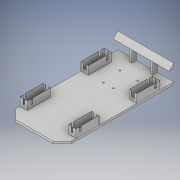
# Autodesk Inventor part: RC Chassis
Saved by Autodesk Inventor 2019 (Build 230136000, 136)
## iProperties
Created: 2020-11-23
Part Number: RC Chassis
Material: Generic
Document SubType Name: Modeling
Designer: wrong
Density: 1 g/cm^3
Appearance: Default
Author: wrong
Autodesk Inventor part; units mm, degrees
ref_plane "YZ Plane" through (0, 0, 0) normal (1, 0, 0) x (0, 1, 0)
sketch "Sketch1" plane through (0, 0, 0) normal (0, 1, 0) x (-1, 0, 0)
  line L0 (0, 0) -> (152.4, 0)
  line L1 (152.4, 0) -> (152.4, 304.8)
  line L2 (152.4, 304.8) -> (0, 304.8)
  line L3 (0, 304.8) -> (0, 0)
  dimension "d0" = 152.4
  dimension "d1" = 304.8
  constraints: 8 end point, 2 parallel, 1 horizontal, 1 perpendicular
  measures "d0" distance of L2.end L1.end
  measures "d1" distance of L1.end L0.end
extrude "Extrusion1" add sketch "Sketch1" along normal blind 50.8
sketch "Sketch3" plane through (0, 50.8, 0) normal (0, 1, 0) x (1, 0, 0)
  line L0 (-152.4, -12.7) -> (0, -12.7)
  line L1 (0, -12.7) -> (0, -304.8)
  line L2 (0, -304.8) -> (-152.4, -304.8)
  line L3 (-152.4, -304.8) -> (-152.4, -12.7)
  line L4 (0, 0) -> (-152.4, 0) projected
  line L5 (0, -304.8) -> (0, 0) projected
  dimension "d8" = 12.7
  dimension "d9" = 152.4
  dimension "d10" = 0
  dimension "d11" = 292.1
  constraints: 8 end point, 2 parallel, 1 horizontal, 1 perpendicular
  measures "d8" distance between parallel lines of L4 L0
  measures "d9" distance of L1.end L2.end
  measures "d10" distance between parallel lines of L5 L1
  measures "d11" distance of L2.end L0.start
extrude "Extrusion2" cut sketch "Sketch3" against normal blind 44.45
sketch "Sketch4" plane through (-152.4, 50.8, 12.7) normal (0, 0, 1) x (1, 0, 0)
  line L0 (10.16, -44.45) -> (0, -44.45)
  line L1 (107.95, -12.7) -> (101.6, -12.7)
  line L2 (101.6, -12.7) -> (101.6, -44.45)
  line L3 (101.6, -44.45) -> (107.95, -44.45)
  line L4 (107.95, -44.45) -> (107.95, -12.7)
  line L5 (152.4, 0) -> (152.4, -44.45) projected
  line L6 (0, 0) -> (152.4, 0) projected
  line L7 (152.4, -44.45) -> (0, -44.45) projected
  line L8 (44.45, -12.7) -> (50.8, -12.7)
  line L9 (50.8, -12.7) -> (50.8, -44.45)
  line L10 (50.8, -44.45) -> (44.45, -44.45)
  line L11 (44.45, -44.45) -> (44.45, -12.7)
  line L12 (0, -44.45) -> (0, 0) projected
  line L13 (44.45, -12.7) -> (0, -12.7)
  line L14 (44.45, -12.7) -> (152.4, -12.7)
  point P0 (152.4, -50.8)
  dimension "d15" = 44.45
  dimension "d16" = 6.35
  dimension "d18" = 31.75
  dimension "d22" = 0
  dimension "d23" = 6.35
  dimension "d24" = 31.75
  dimension "d25" = 44.45
  constraints: 22 end point, 4 parallel, 4 point on line, 3 horizontal, 2 perpendicular
  measures "d15" distance between parallel lines of L5 L4
  measures "d16" distance of L1.start L1.end
  measures "d18" distance of L1.end L2.end
  measures "d22" distance between parallel lines of L7 L3
  measures "d23" distance of L8.start L8.end
  measures "d24" distance of L10.end L8.start
  measures "d25" distance between parallel lines of L12 L11
extrude "Extrusion3" cut sketch "Sketch4" against normal through all contours L0 L12 L13 L11 L7 | L9 L14 L2 L7 | L4 L14 L5 L7
chamfer "Chamfer1" distance 12.7 angle 45 1 edges at (-76.2, 50.8, 12.7)
chamfer "Chamfer2" distance 25.4 angle 45 2 edges at (-152.4, 3.175, 304.8) (0, 3.175, 304.8) measured on face at (-101.6, 2.1167, 304.8)
sketch "Sketch8" plane through (0, 6.35, 0) normal (0, 1, 0) x (1, 0, 0)
  line L0 (-102.7176, -33.0495) -> (-49.7078, -33.0495)
  line L1 (-49.7078, -33.0495) -> (-49.7078, -100.3087)
  line L2 (-49.7078, -100.3087) -> (-102.7176, -100.3087)
  line L3 (-102.7176, -100.3087) -> (-102.7176, -33.0495)
  circle A0 centre (-94.0562, -97.3877) radius 1.9939
  circle A1 centre (-67.056, -97.3877) radius 1.9939
  circle A2 centre (-100.5078, -46.4861) radius 1.9939
  circle A3 centre (-51.9176, -46.4861) radius 1.9939
  line L4 (-25.3492, -49.0474) -> (-25.3492, -97.3582) projected
  line L5 (-67.056, -97.3877) -> (-51.9176, -97.3877)
  point P0 (0, 0)
  dimension "d72" = 53.0098
  dimension "d73" = 67.2592
  dimension "d74" = 3.9878
  dimension "d75" = 2.921
  dimension "d76" = 8.6614
  dimension "d77" = 3.9878
  dimension "d78" = 27.0002
  dimension "d79" = 3.9878
  dimension "d81" = 2.2098
  dimension "d84" = 3.9878
  dimension "d85" = 2.2098
  dimension "d87" = 24.3586
  dimension "d99" = 50.9016
  dimension "d100" = 13.4366
  dimension "d101" = 13.4366
  constraints: 10 end point, 4 centre point, 2 horizontal, 2 parallel, 1 perpendicular
  measures "d72" distance of L1.end L2.end
  measures "d73" distance of L0.end L1.end
  measures "d74" diameter of A0
  measures "d75" distance from line of L2 A0.centre
  measures "d76" distance from line of L3 A0.centre
  measures "d77" diameter of A1
  measures "d78" distance of L5.start A0.centre
  measures "d79" diameter of A2
  measures "d81" distance from line of L3 A2.centre
  measures "d84" diameter of A3
  measures "d85" distance from line of L1 A3.centre
  measures "d87" distance between parallel lines of L1 L4
  measures "d99" distance from line of A3.centre L5
  measures "d100" distance from line of L0 A3.centre
  measures "d101" distance from line of L0 A2.centre
hole "Hole1" at (-94.0562, 6.35, 97.3877) at (-67.056, 6.35, 97.3877) at (-100.5078, 6.35, 46.4861) at (-51.9176, 6.35, 46.4861) direction (0, -1, 0) diameter 3.9878 end through all
sketch "Sketch11" plane through (0, 6.35, 0) normal (0, 1, 0) x (1, 0, 0)
  line L0 (-143.515, -33.715) -> (-143.515, -38.215) projected
  line L1 (-141.015, -33.715) -> (-141.015, -38.215) projected
  line L2 (-143.515, -33.215) -> (-141.015, -33.215) projected
  line L3 (-142.265, -75.215) -> (-133.265, -75.215) projected
  line L4 (-133.265, -75.215) -> (-133.265, -43.215) projected
  line L5 (-133.265, -43.215) -> (-151.265, -43.215) projected
  line L6 (-151.265, -43.215) -> (-151.265, -75.215) projected
  line L7 (-151.265, -75.215) -> (-142.265, -75.215) projected
  line L8 (-151.265, -38.215) -> (-133.265, -38.215) projected
  line L9 (-160.765, -52.415) -> (-123.765, -52.415)
  line L10 (-160.765, -47.015) -> (-123.765, -47.015)
  line L11 (-150.565, -75.215) -> (-150.565, -86.215) projected
  line L12 (-149.165, -100.215) -> (-143.2099, -100.215) projected
  line L13 (-141.3201, -100.215) -> (-135.365, -100.215) projected
  line L14 (-146.165, -102.415) -> (-137.365, -102.415) projected
  arc A0 (-132.765, -38.715) -> (-133.265, -38.215) centre (-133.265, -38.715) ccw projected
  arc A1 (-151.265, -38.215) -> (-151.765, -38.715) centre (-151.265, -38.715) ccw projected
  line L15 (-151.765, -38.715) -> (-151.765, -43.215) projected
  line L16 (-132.765, -43.215) -> (-132.765, -38.715) projected
  line L17 (-143.015, -103.215) -> (-141.515, -103.215) projected
  line L18 (-152.019, -37.961) -> (-132.511, -37.961)
  line L19 (-132.511, -37.961) -> (-132.511, -100.469)
  line L20 (-132.511, -100.469) -> (-152.019, -100.469)
  line L21 (-152.019, -100.469) -> (-152.019, -37.961)
  line L22 (-152.4, -279.4) -> (-152.4, 0) projected
  line L23 (-152.4, -37.58) -> (-132.13, -37.58)
  line L24 (-132.13, -37.58) -> (-132.13, -100.85)
  line L25 (-132.13, -100.85) -> (-152.4, -100.85)
  line L26 (-152.4, -100.85) -> (-152.4, -37.58)
  line L27 (-76.2, -26.595) -> (-76.2, -134.8867)
  line L28 (0, 0) -> (0, -279.4) projected
  line L29 (-19.889, -37.961) -> (-19.889, -100.469)
  dimension "d102" = 0.254
  dimension "d103" = 0.254
  dimension "d104" = 0.254
  dimension "d105" = 0.254
  dimension "d106" = 0.381
  dimension "d107" = 0.381
  dimension "d108" = 0.381
  dimension "d115" = 76.2
  constraints: 24 end point, 4 horizontal, 4 parallel, 2 perpendicular, 2 symmetric about line, 1 point on line, 1 vertical, 4 other
  measures "d102" distance between parallel lines of L19 L16
  measures "d103" distance between parallel lines of L15 L21
  measures "d104" distance between parallel lines of L8 L18
  measures "d105" distance between parallel lines of L12 L20
  measures "d106" distance between parallel lines of L18 L23
  measures "d107" distance between parallel lines of L19 L24
  measures "d108" distance between parallel lines of L20 L25
  measures "d115" distance between parallel lines of L28 L27
extrude "Extrusion6" add sketch "Sketch11" along normal blind 22.5044 contours L23 L1 L18 L0 | L0 L18 L21 L10 L22 L23 | L23 L24 L10 L19 L18 L1 | L10 L21 L9 L22 | L9 L21 L20 L19 L24 L25 L22 | L24 L9 L19 L10
sketch "Sketch13" plane through (-132.13, 6.35, 100.85) normal (1, 0, 0) x (0, 0, -1)
  circle A0 centre (51.135, 11.25) radius 2.8 projected
  line L0 (48.3356, 11.3067) -> (48.3356, 22.5044)
  line L1 (0, 22.5044) -> (63.27, 22.5044) projected
  line L2 (48.3356, 11.3067) -> (59.5333, 11.3067) construction
  line L3 (53.9344, 11.3067) -> (53.9344, 22.5044)
  line L4 (53.9344, 11.3067) -> (65.1321, 11.3067) construction
  line L5 (48.3356, 22.5044) -> (53.9344, 22.5044)
  arc A1 (48.3356, 11.3067) -> (53.9344, 11.3067) centre (51.135, 11.25) ccw
  point P0 (100.85, -6.35)
  dimension "d111" = 90
  dimension "d112" = 90
  constraints: 10 end point, 2 horizontal, 2 midpoint, 2 perpendicular, 2 point on circle, 2 point on line, 1 centre point, 1 coincident, 1 collinear, 3 other
  measures "d111" angle of L2 L0
  measures "d112" angle of L4 L3
extrude "Extrusion7" cut sketch "Sketch13" against normal through all
sketch "Sketch14" plane through (-152.4, 6.35, 100.85) normal (0, 0, 1) x (1, 0, 0)
  arc A0 (6.235, 8.2835) -> (6.235, 14.2165) centre (10.135, 11.25) ccw projected
  line L0 (6.235, 14.2165) -> (6.235, 8.2835) projected
  line L1 (5.981, 8.7157) -> (5.981, 13.3615)
  line L2 (0, 22.5044) -> (20.27, 22.5044) projected
  line L3 (5.981, 13.3615) -> (5.981, 22.5044)
  line L4 (15.289, 22.5044) -> (5.981, 22.5044)
  arc A1 (6.235, 8.2835) -> (5.981, 13.8489) centre (10.135, 11.25) ccw
  line L5 (15.035, 11.25) -> (15.035, 22.5044)
  line L6 (19.889, 22.5044) -> (0.381, 22.5044) projected
  line L7 (15.035, 11.25) -> (26.2894, 11.25) construction
  point P0 (152.4, -6.35)
  dimension "d116" = 0.254
  dimension "d118" = 90
  constraints: 11 end point, 4 point on circle, 4 point on line, 2 perpendicular, 1 centre point, 1 coincident, 1 concentric, 1 horizontal, 1 parallel
  measures "d116" distance between parallel lines of L0 L1
  measures "d118" angle of L7 L5
ref_plane "Work Plane1" through (-76.2, 0, 0) normal (1, 0, 0) x (0, 0, -1)
ref_plane "Work Plane2" through (-127, 0, 152.4) normal (0, 0, 1) x (1, 0, 0)
extrude "Extrusion8" cut sketch "Sketch14" against normal up to surface (0.381 mm away)
sketch "Sketch15" plane through (-132.13, 6.35, 37.58) normal (0, 0, -1) x (-1, 0, 0)
  line L0 (8.885, 13.25) -> (8.885, 9.25) projected
  line L1 (11.385, 9.25) -> (11.385, 13.25) projected
  line L2 (11.385, 8.75) -> (8.885, 8.75) projected
  line L3 (0, 22.5044) -> (20.27, 22.5044) projected
  line L4 (8.631, 8.75) -> (8.631, 22.5044)
  line L5 (19.889, 22.5044) -> (0.381, 22.5044) projected
  line L6 (11.639, 8.75) -> (11.639, 22.5044)
  line L7 (8.631, 22.5044) -> (11.639, 22.5044)
  line L8 (8.631, 8.75) -> (8.885, 8.75)
  line L9 (11.385, 8.75) -> (11.639, 8.75)
  line L10 (8.885, 8.75) -> (11.385, 8.75)
  point P0 (-132.13, -6.35)
  dimension "d121" = 0.254
  dimension "d122" = 0.254
  constraints: 12 end point, 3 collinear, 2 perpendicular, 2 point on line, 1 parallel
  measures "d121" distance between parallel lines of L0 L4
  measures "d122" distance between parallel lines of L1 L6
extrude "Extrusion9" cut sketch "Sketch15" against normal up to surface (0.381 mm away)
mirror "Mirror2" about plane through (-127, 0, 152.4) normal (0, 0, 1) of "Extrusion6", "Extrusion7", "Extrusion8", "Extrusion9"
mirror "Mirror3" about plane through (-76.2, 0, 0) normal (1, 0, 0) of "Extrusion6", "Extrusion7", "Extrusion8", "Extrusion9", "Mirror2"
body "Solid1"
